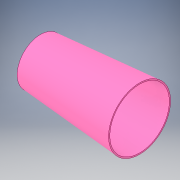
# Autodesk Inventor part: boues
Saved by Autodesk Inventor 2019 (Build 230136000, 136)
## iProperties
Created: 2020-02-15
Part Number: boues
Material: Generic
Document SubType Name: Modeling
Designer: franc
Density: 1 g/cm^3
Appearance: Default
Author: franc
Autodesk Inventor part; units mm, degrees
ref_plane "YZ Plane" through (0, 0, 0) normal (1, 0, 0) x (0, 1, 0)
ref_plane "XZ Plane" through (0, 0, 0) normal (0, 1, 0) x (-1, 0, 0)
ref_plane "XY Plane" through (0, 0, 0) normal (0, 0, 1) x (1, 0, 0)
sketch "Esquisse1" plane through (0, 0, 0) normal (0, 1, 0) x (-1, 0, 0)
  line L0 (56.3598, 0) -> (-58.6402, 0)
  line L1 (-58.6402, -34.5) -> (-58.6402, -36)
  line L2 (-58.6402, -36) -> (56.3598, -27)
  line L3 (56.3598, -27) -> (56.3598, 0)
  line L4 (54.8598, 0) -> (54.8598, -25.6128)
  line L5 (54.8598, -25.6128) -> (-58.6402, -34.5)
  point P0 (0, 0)
  dimension "d0" = 115
  dimension "d1" = 27
  dimension "d2" = 36
  dimension "d3" = 1.5
  dimension "d4" = 1.5
  dimension "d5" = 1.5
  constraints: 12 end point, 1 horizontal, 1 parallel, 1 perpendicular, 1 point on line, 1 vertical
  measures "d0" distance of L0.start L0.end
  measures "d1" distance of L2.end L0.start
  measures "d2" distance of L0.end L1.end
  measures "d3" distance between parallel lines of L3 L4
  measures "d4" distance of L1.start L1.end
  measures "d5" distance from line of L2 L4.end
revolve "Révolution1" add sketch "Esquisse1" angle 360 about axis through (-56.3598, 0, 0) along (1, 0, 0)
